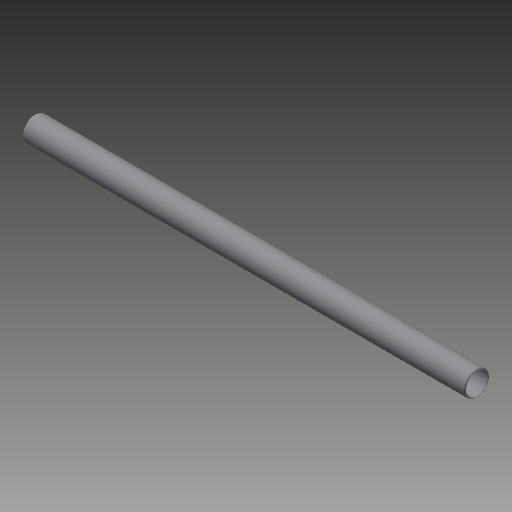
# Autodesk Inventor part: 12R-23.48650SR
Saved by Autodesk Inventor 2019 (Build 230136000, 136)
## iProperties
Category: PARTsolutions
Company: BIMBA
Created: 2019-01-13
Part Number: 12R-23.48650SR
Material: Generic
Catalog Web Link: www.cadenas.de
Description: Tube-Original Line - Standard Air Cylinders
Vendor: BIMBA
Document SubType Name: Modeling
Designer: psadmin
Manufacturer: BIMBA
Mass: 51.0885 g
Surface Area: 1237.84 cm^2
Volume: 51.0885 cm^3
Density: 1 g/cm^3
Appearance: PSOLRGB-180-180-180
PSOL_IDENT_0: {$CADENAS_DATA\23d-libs\bimba\bimba\bimba_imperial\bimba_full_line\original_line_cylinders\standard_
PSOL_IDENT_1: air_cylinders\tube.prj},205 {VTYP=3D},{NB=12R-23.48650SR},{LINA=12R-23.48650SR},{NN=Tube},{DATE=21.0
PSOL_IDENT_2: 3.2018 14:31:21},{GEOMDATE=18.02.2011 00:00:00},{VERSION=},{LINEID=70},{WBVAR=MNT,ACTING,NR,L,FOURHO
PSOL_IDENT_3: LES,SR},{WBNUMERIC=L,FOURHOLES}  {NB=12R-23.48650SR},{LINA=12R-23.48650SR},{KT=DUMMY},{PN=12R-23.486
PSOL_IDENT_4: 50SR},{BORE=1.25000000},{BOREPN=12},{MNT=},{MNTALG='' , 'Front Nose'},{ACTING=R},{ACTINGALG= '' , 'S
PSOL_IDENT_5: ingle Acting' , 'R' , 'Reverse/Double Acting' },{NR=},{NRALG= '' , 'N/A' },{L=23.4865},{OD=1.3265},{
PSOL_IDENT_6: ODN=1.3265},{ODP=1.3265},{ODB=0.0000},{ID=1.2615},{DV=0.00000000},{LV=0.00000000},{LV1=0.00000000},{
PSOL_IDENT_7: G=0.0400},{FOURHOLES=0},{AA=0.3750},{BB=0.0940},{SR=SR},{SRALG= 'C' , 'Carbon Steel Rod' , 'SR' , '3
PSOL_IDENT_8: 03 Stainless Steel Rod' , '' , '303 Stainless Steel Rod'}
NN: Tube
NT: Original Line - Standard Air Cylinders
NB: 12R-23.48650SR
NBSYN: $PN.
LINA: 12R-23.48650SR
BORE: 0
BOREPN: 12
MNT: Front Nose
MNTALG: '' , 'Front Nose'
ACTING: Reverse/Double Acting
NR: N/A
L: 23.4865
ODN: 1.3265
ODP: 1.3265
ODB: 0
ID: 1.2615
DV: 0
LV: 0
LV1: 0
G: 0.04
FOURHOLES: 0
AA: 0.375
BB: 0.094
SR: 303 Stainless Steel Rod
SUPPLIER: BIMBA
ARTICLENO: 12R-23.48650SR
BOMINFO: 12R-23.48650SR
CREATOR: CADENAS GmbH
Title: 12R-23.48650SR
Author: Cadenas PARTsolutions
Comments: Original Line - Standard Air Cylinders
Autodesk Inventor part; units mm, degrees
sketch "Sketch_1" plane through (0, 0, 0) normal (0, 0, 1) x (1, 0, 0)
  line L0 (596.5571, 0) -> (0, 0)
  arc A0 (-0.8826, 15.5593) -> (-0.8826, 15.3797) centre (-0.7928, 15.4695) ccw
  line L1 (-0.8826, 15.3797) -> (-0.508, 15.0051)
  line L2 (-0.508, 15.0051) -> (0, 15.0051)
  line L3 (0, 15.0051) -> (1.016, 16.021)
  line L4 (1.016, 16.021) -> (595.5411, 16.021)
  line L5 (595.5411, 16.021) -> (596.5571, 15.0051)
  line L6 (596.5571, 15.0051) -> (597.0651, 15.0051)
  line L7 (597.0651, 15.0051) -> (597.4397, 15.3797)
  arc A1 (597.4397, 15.3797) -> (597.4397, 15.5593) centre (597.3499, 15.4695) ccw
  line L8 (597.4397, 15.5593) -> (596.45, 16.549)
  arc A2 (596.45, 16.549) -> (595.7316, 16.8466) centre (595.7316, 15.8305) ccw
  line L9 (595.7316, 16.8466) -> (0.8255, 16.8466)
  arc A3 (0.8255, 16.8466) -> (0.1071, 16.549) centre (0.8255, 15.8305) ccw
  line L10 (0.1071, 16.549) -> (-0.8826, 15.5593)
  constraints: 22 end point, 8 point on circle, 4 centre point
revolve "Revolution1" add sketch "Sketch_1" angle 360 about axis through (596.5571, 0, 0) along (1, 0, 0)
ref_plane "cp1_XY" through (298.2785, 16.8466, 0) normal (1, 0, 0) x (0, 0, -1)
ref_plane "cp1_YZ" through (298.2785, 16.8466, 0) normal (0, 0, -1) x (0, 1, 0)
ref_plane "cp1_ZX" through (298.2785, 16.8466, 0) normal (0, 1, 0) x (1, 0, 0)
ref_plane "cp2_XY" through (298.2785, 0, -16.8466) normal (1, 0, 0) x (0, 0, -1)
ref_plane "cp2_YZ" through (298.2785, 0, -16.8466) normal (0, 0, -1) x (0, 1, 0)
ref_plane "cp2_ZX" through (298.2785, 0, -16.8466) normal (0, 1, 0) x (1, 0, 0)
ref_plane "cp3_XY" through (298.2785, -16.8466, 0) normal (1, 0, 0) x (0, 0, -1)
ref_plane "cp3_YZ" through (298.2785, -16.8466, 0) normal (0, 0, -1) x (0, 1, 0)
ref_plane "cp3_ZX" through (298.2785, -16.8466, 0) normal (0, 1, 0) x (1, 0, 0)
ref_plane "cp4_XY" through (298.2785, 0, 16.8466) normal (1, 0, 0) x (0, 0, -1)
ref_plane "cp4_YZ" through (298.2785, 0, 16.8466) normal (0, 0, -1) x (0, 1, 0)
ref_plane "cp4_ZX" through (298.2785, 0, 16.8466) normal (0, 1, 0) x (1, 0, 0)
ref_plane "tube_front_XY" through (0, 0, 0) normal (1, 0, 0) x (0, 0, -1)
ref_plane "tube_front_YZ" through (0, 0, 0) normal (0, 0, -1) x (0, 1, 0)
ref_plane "tube_front_ZX" through (0, 0, 0) normal (0, 1, 0) x (1, 0, 0)
ref_plane "tube_rear_XY" through (596.5571, 0, 0) normal (1, 0, 0) x (0, 0, -1)
ref_plane "tube_rear_YZ" through (596.5571, 0, 0) normal (0, 0, -1) x (0, 1, 0)
ref_plane "tube_rear_ZX" through (596.5571, 0, 0) normal (0, 1, 0) x (1, 0, 0)
body "Solid1"
